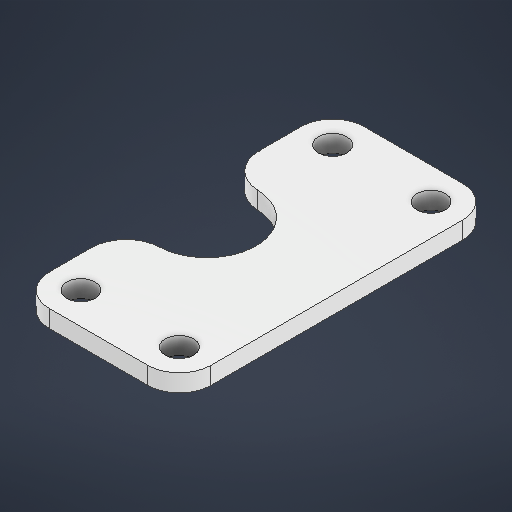
# Autodesk Inventor part: CNC-002-ShimStructureGusset2
Saved by Autodesk Inventor 2026.2 (Build 302298000, 298)
## iProperties
Created: 2026-06-14
Part Number: CNC-002-ShimStructureGusset2
Material: ABS Plastic
Document SubType Name: Modeling
Designer: Kenji
Density: 1.06 g/cm^3
Appearance: Smooth - White
Author: Kenji
Autodesk Inventor part; units mm, degrees
ref_plane "YZ Plane" through (0, 0, 0) normal (1, 0, 0) x (0, 1, 0)
ref_plane "XZ Plane" through (0, 0, 0) normal (0, 1, 0) x (-1, 0, 0)
ref_plane "XY Plane" through (0, 0, 0) normal (0, 0, 1) x (1, 0, 0)
sketch "Sketch1" plane through (0, 0, 0) normal (0, 1, 0) x (-1, 0, 0)
  circle A0 centre (0, 0) radius 2.6
  circle A1 centre (-18, 0) radius 2.6
  circle A2 centre (0, -46) radius 2.6
  circle A3 centre (-18, -46) radius 2.6
  circle A4 centre (0, -23) radius 9 construction
  circle A5 centre (0, 0) radius 5.775 construction
  circle A6 centre (0, -46) radius 5.775 construction
  circle A7 centre (-18, -46) radius 5.775 construction
  circle A8 centre (-18, 0) radius 5.775 construction
  line L0 (5.775, 0) -> (5.775, -7.6608)
  line L1 (5.775, -46) -> (5.775, -38.3392)
  arc A9 (5.775, -38.3392) -> (-0.3371, -31.9937) centre (-0.575, -38.3392) ccw
  arc A10 (-0.3371, -14.0063) -> (5.775, -7.6608) centre (-0.575, -7.6608) ccw
  arc A11 (-0.3371, -14.0063) -> (-0.3371, -31.9937) centre (0, -23) ccw
  line L2 (-23.775, 0) -> (-23.775, -46)
  line L3 (0, -51.775) -> (-18, -51.775)
  line L4 (0, 5.775) -> (-18, 5.775)
  arc A12 (5.775, 0) -> (0, 5.775) centre (0, 0) ccw
  arc A13 (-18, 5.775) -> (-23.775, 0) centre (-18, 0) ccw
  arc A14 (0, -51.775) -> (5.775, -46) centre (0, -46) ccw
  arc A15 (-23.775, -46) -> (-18, -51.775) centre (-18, -46) ccw
  dimension "d0" = 5.2
  dimension "d1" = 18
  dimension "d2" = 46
  dimension "d3" = 18
  dimension "d4" = 23
  dimension "d5" = 3.175
  dimension "d6" = 6.35
  constraints: 24 point on circle, 16 centre point, 11 equal radius, 11 tangent, 10 end point, 4 coincident, 3 vertical, 3 vertical alignment, 2 horizontal, 2 horizontal alignment
  measures "d0" diameter of A0
  measures "d1" distance of A1.centre point (0, 0)
  measures "d2" distance of A1.centre A3.centre
  measures "d3" diameter of A4
  measures "d4" distance of A4.centre point (0, 0)
  measures "d5" radial gap between concentric circles of A5 A0
  measures "d6" radius of A9
extrude "Extrusion1" add sketch "Sketch1" along normal blind 3.175
equation "\"d4\" = 0.5 * d2"
body "Solid1"
